Autodesk Inventor part; units mm, degrees
(part 2 of 2)
  arc A454 (149.024, -44.4083) -> (153.7778, -44.1859) centre (149.9853, -14.0418) ccw projected
  arc A455 (153.7778, -44.1859) -> (154.2042, -42.674) centre (0, 0) ccw projected
  arc A456 (154.2042, -42.674) -> (150.2671, -40.0005) centre (135.2203, -66.3945) ccw projected
  arc A457 (150.2671, -40.0005) -> (150.6526, -38.5234) centre (0, 0) ccw projected
  arc A458 (150.6526, -38.5234) -> (155.394, -38.1145) centre (150.4209, -8.1425) ccw projected
  arc A459 (155.394, -38.1145) -> (155.7607, -36.5871) centre (0, 0) ccw projected
  arc A460 (155.7607, -36.5871) -> (151.7217, -34.0702) centre (137.7226, -61.0346) ccw projected
  arc A461 (151.7217, -34.0702) -> (152.0488, -32.5791) centre (0, 0) ccw projected
  arc A462 (152.0488, -32.5791) -> (156.7705, -31.9844) centre (150.6246, -2.2308) ccw projected
  arc A463 (156.7705, -31.9844) -> (157.077, -30.4438) centre (0, 0) ccw projected
  arc A464 (157.077, -30.4438) -> (152.9423, -28.0874) centre (140.0127, -55.5806) ccw projected
  arc A465 (152.9423, -28.0874) -> (153.2107, -26.5846) centre (0, 0) ccw projected
  arc A466 (153.2107, -26.5846) -> (157.9054, -25.8049) centre (150.5961, 3.6845) ccw projected
  arc A467 (157.9054, -25.8049) -> (158.1511, -24.2535) centre (0, 0) ccw projected
  arc A468 (158.1511, -24.2535) -> (153.9271, -22.0613) centre (142.0868, -50.0409) ccw projected
  arc A469 (153.9271, -22.0613) -> (154.1363, -20.5491) centre (0, 0) ccw projected
  arc A470 (154.1363, -20.5491) -> (158.7967, -19.5857) centre (150.3353, 9.594) ccw projected
  arc A471 (158.7967, -19.5857) -> (158.9814, -18.0258) centre (0, 0) ccw projected
  arc A472 (158.9814, -18.0258) -> (154.6745, -16.0011) centre (143.9419, -44.424) ccw projected
  arc A473 (154.6745, -16.0011) -> (154.8242, -14.4819) centre (0, 0) ccw projected
  arc A474 (154.8242, -14.4819) -> (159.4432, -13.3363) centre (149.8427, 15.4887) ccw projected
  arc A475 (159.4432, -13.3363) -> (159.5665, -11.7703) centre (0, 0) ccw projected
  arc A476 (159.5665, -11.7703) -> (155.1835, -9.9163) centre (145.575, -38.7386) ccw projected
  arc A477 (155.1835, -9.9163) -> (155.2734, -8.3923) centre (0, 0) ccw projected
  arc A478 (155.2734, -8.3923) -> (159.8439, -7.0663) centre (149.1191, 21.3596) ccw projected
  arc A479 (159.8439, -7.0663) -> (159.9056, -5.4967) centre (0, 0) ccw projected
  arc A480 (159.9056, -5.4967) -> (155.4532, -3.8162) centre (146.9836, -32.9935) ccw projected
  arc A481 (155.4532, -3.8162) -> (155.4831, -2.2898) centre (0, 0) ccw projected
  arc A482 (155.4831, -2.2898) -> (159.9981, -0.7854) centre (148.1656, 27.1975) ccw projected
  arc A483 (159.9981, -0.7854) -> (159.9981, 0.7854) centre (0, 0) ccw projected
  arc A484 (159.9981, 0.7854) -> (155.4831, 2.2898) centre (148.1656, -27.1975) ccw projected
  arc A485 (155.4831, 2.2898) -> (155.4532, 3.8162) centre (0, 0) ccw projected
  arc A486 (155.4532, 3.8162) -> (159.9056, 5.4967) centre (146.9836, 32.9935) ccw projected
  arc A487 (159.9056, 5.4967) -> (159.8439, 7.0663) centre (0, 0) ccw projected
  arc A488 (159.8439, 7.0663) -> (155.2734, 8.3923) centre (149.1191, -21.3596) ccw projected
  arc A489 (155.2734, 8.3923) -> (155.1835, 9.9163) centre (0, 0) ccw projected
  arc A490 (155.1835, 9.9163) -> (159.5665, 11.7703) centre (145.575, 38.7386) ccw projected
  arc A491 (159.5665, 11.7703) -> (159.4432, 13.3363) centre (0, 0) ccw projected
  arc A492 (159.4432, 13.3363) -> (154.8242, 14.4819) centre (149.8427, -15.4887) ccw projected
  arc A493 (154.8242, 14.4819) -> (154.6745, 16.0011) centre (0, 0) ccw projected
  arc A494 (154.6745, 16.0011) -> (158.9814, 18.0258) centre (143.9419, 44.424) ccw projected
  arc A495 (158.9814, 18.0258) -> (158.7967, 19.5857) centre (0, 0) ccw projected
  arc A496 (158.7967, 19.5857) -> (154.1363, 20.5491) centre (150.3353, -9.594) ccw projected
  arc A497 (154.1363, 20.5491) -> (153.9271, 22.0613) centre (0, 0) ccw projected
  arc A498 (153.9271, 22.0613) -> (158.1511, 24.2535) centre (142.0868, 50.0409) ccw projected
  arc A499 (158.1511, 24.2535) -> (157.9054, 25.8049) centre (0, 0) ccw projected
  arc A500 (157.9054, 25.8049) -> (153.2107, 26.5846) centre (150.5961, -3.6845) ccw projected
  arc A501 (153.2107, 26.5846) -> (152.9423, 28.0874) centre (0, 0) ccw projected
  arc A502 (152.9423, 28.0874) -> (157.077, 30.4438) centre (140.0127, 55.5806) ccw projected
  arc A503 (157.077, 30.4438) -> (156.7705, 31.9844) centre (0, 0) ccw projected
  arc A504 (156.7705, 31.9844) -> (152.0488, 32.5791) centre (150.6246, 2.2308) ccw projected
  arc A505 (152.0488, 32.5791) -> (151.7217, 34.0702) centre (0, 0) ccw projected
  arc A506 (151.7217, 34.0702) -> (155.7607, 36.5871) centre (137.7226, 61.0346) ccw projected
  arc A507 (155.7607, 36.5871) -> (155.394, 38.1145) centre (0, 0) ccw projected
  arc A508 (155.394, 38.1145) -> (150.6526, 38.5234) centre (150.4209, 8.1425) ccw projected
  arc A509 (150.6526, 38.5234) -> (150.2671, 40.0005) centre (0, 0) ccw projected
  arc A510 (150.2671, 40.0005) -> (154.2042, 42.674) centre (135.2203, 66.3945) ccw projected
  arc A511 (154.2042, 42.674) -> (153.7778, 44.1859) centre (0, 0) ccw projected
  arc A512 (153.7778, 44.1859) -> (149.024, 44.4083) centre (149.9853, 14.0418) ccw projected
  arc A513 (149.024, 44.4083) -> (148.5809, 45.8692) centre (0, 0) ccw projected
  arc A514 (148.5809, 45.8692) -> (152.4099, 48.6952) centre (132.5094, 71.6521) ccw projected
  arc A515 (152.4099, 48.6952) -> (151.9245, 50.1891) centre (0, 0) ccw projected
  arc A516 (151.9245, 50.1891) -> (147.1657, 50.2247) centre (149.3183, 19.9193) ccw projected
  arc A517 (147.1657, 50.2247) -> (146.6655, 51.6671) centre (0, 0) ccw projected
  arc A518 (146.6655, 51.6671) -> (150.3806, 54.6412) centre (129.5942, 76.7991) ccw projected
  arc A519 (150.3806, 54.6412) -> (149.837, 56.1149) centre (0, 0) ccw projected
  arc A520 (149.837, 56.1149) -> (145.0804, 55.9637) centre (148.4212, 25.7662) ccw projected
  arc A521 (145.0804, 55.9637) -> (144.524, 57.3853) centre (0, 0) ccw projected
  arc A522 (144.524, 57.3853) -> (148.1195, 60.503) centre (126.4791, 81.8277) ccw projected
  arc A523 (148.1195, 60.503) -> (147.5184, 61.9542) centre (0, 0) ccw projected
  arc A524 (147.5184, 61.9542) -> (142.7714, 61.6164) centre (147.2952, 31.5733) ccw projected
  arc A525 (142.7714, 61.6164) -> (142.1596, 63.015) centre (0, 0) ccw projected
  arc A526 (142.1596, 63.015) -> (145.63, 66.2715) centre (123.1691, 86.7302) ccw projected
  arc A527 (145.63, 66.2715) -> (144.9723, 67.698) centre (0, 0) ccw projected
  arc A528 (144.9723, 67.698) -> (140.2423, 67.174) centre (145.9421, 37.3317) ccw projected
  arc A529 (140.2423, 67.174) -> (139.5761, 68.5476) centre (0, 0) ccw projected
  arc A530 (139.5761, 68.5476) -> (142.9159, 71.9378) centre (119.6691, 91.4989) ccw projected
  arc A531 (142.9159, 71.9378) -> (142.2028, 73.3374) centre (0, 0) ccw projected
  arc A532 (142.2028, 73.3374) -> (137.4969, 72.6281) centre (144.3639, 43.0326) ccw projected
  arc A533 (137.4969, 72.6281) -> (136.7773, 73.9745) centre (0, 0) ccw projected
  arc A534 (136.7773, 73.9745) -> (139.9814, 77.4932) centre (115.9846, 96.1266) ccw projected
  arc A535 (139.9814, 77.4932) -> (139.2139, 78.8637) centre (0, 0) ccw projected
  arc A536 (139.2139, 78.8637) -> (134.5396, 77.9702) centre (142.5632, 48.6671) ccw projected
  arc A537 (134.5396, 77.9702) -> (133.7676, 79.2873) centre (0, 0) ccw projected
  arc A538 (133.7676, 79.2873) -> (136.8312, 82.9291) centre (112.1213, 100.606) ccw projected
  arc A539 (136.8312, 82.9291) -> (136.0104, 84.2684) centre (0, 0) ccw projected
  arc A540 (136.0104, 84.2684) -> (131.3747, 83.1921) centre (140.5426, 54.2266) ccw projected
  arc A541 (131.3747, 83.1921) -> (130.5517, 84.4779) centre (0, 0) ccw projected
  arc A542 (130.5517, 84.4779) -> (133.4699, 88.2371) centre (108.0851, 104.9303) ccw projected
  arc A543 (133.4699, 88.2371) -> (132.5972, 89.5432) centre (0, 0) ccw projected
  arc A544 (132.5972, 89.5432) -> (128.0073, 88.2857) centre (138.3053, 59.7025) ccw projected
  arc A545 (128.0073, 88.2857) -> (127.1344, 89.5382) centre (0, 0) ccw projected
  arc A546 (127.1344, 89.5382) -> (129.9028, 93.4091) centre (103.8822, 109.0928) ccw projected
  arc A547 (129.9028, 93.4091) -> (128.9795, 94.6799) centre (0, 0) ccw projected
  arc A548 (128.9795, 94.6799) -> (124.4426, 93.2432) centre (135.8548, 65.0863) ccw projected
  arc A549 (124.4426, 93.2432) -> (123.5212, 94.4604) centre (0, 0) ccw projected
  arc A550 (123.5212, 94.4604) -> (126.1354, 98.4371) centre (99.5191, 113.0871) ccw projected
  arc A551 (126.1354, 98.4371) -> (125.163, 99.6706) centre (0, 0) ccw projected
  arc A552 (125.163, 99.6706) -> (120.6859, 98.0569) centre (133.1948, 70.3698) ccw projected
  arc A553 (120.6859, 98.0569) -> (119.7174, 99.237) centre (0, 0) ccw projected
  arc A554 (119.7174, 99.237) -> (122.1736, 103.3132) centre (95.0026, 116.907) ccw projected
  arc A555 (122.1736, 103.3132) -> (121.1534, 104.5077) centre (0, 0) ccw projected
  arc A556 (121.1534, 104.5077) -> (116.7432, 102.7194) centre (130.3294, 75.5447) ccw projected
  arc A557 (116.7432, 102.7194) -> (115.7291, 103.8606) centre (0, 0) ccw projected
  arc A558 (115.7291, 103.8606) -> (118.0233, 108.0301) centre (90.3396, 120.5467) ccw projected
  arc A559 (118.0233, 108.0301) -> (116.9571, 109.1835) centre (0, 0) ccw projected
  arc A560 (116.9571, 109.1835) -> (112.6204, 107.2236) centre (127.263, 80.6032) ccw projected
  arc A561 (112.6204, 107.2236) -> (111.5623, 108.324) centre (0, 0) ccw projected
  arc A562 (111.5623, 108.324) -> (113.6911, 112.5804) centre (85.5374, 124.0004) ccw projected
  arc A563 (113.6911, 112.5804) -> (112.5804, 113.6911) centre (0, 0) ccw projected
  arc A564 (112.5804, 113.6911) -> (108.324, 111.5623) centre (124.0004, 85.5374) ccw projected
  arc A565 (108.324, 111.5623) -> (107.2236, 112.6204) centre (0, 0) ccw projected
  arc A566 (107.2236, 112.6204) -> (109.1835, 116.9571) centre (80.6032, 127.263) ccw projected
  arc A567 (109.1835, 116.9571) -> (108.0301, 118.0233) centre (0, 0) ccw projected
  arc A568 (108.0301, 118.0233) -> (103.8606, 115.7291) centre (120.5467, 90.3396) ccw projected
  arc A569 (103.8606, 115.7291) -> (102.7194, 116.7432) centre (0, 0) ccw projected
  arc A570 (102.7194, 116.7432) -> (104.5077, 121.1534) centre (75.5447, 130.3294) ccw projected
  arc A571 (104.5077, 121.1534) -> (103.3132, 122.1736) centre (0, 0) ccw projected
  arc A572 (103.3132, 122.1736) -> (99.237, 119.7174) centre (116.907, 95.0026) ccw projected
  arc A573 (99.237, 119.7174) -> (98.0569, 120.6859) centre (0, 0) ccw projected
  arc A574 (98.0569, 120.6859) -> (99.6706, 125.163) centre (70.3698, 133.1948) ccw projected
  arc A575 (99.6706, 125.163) -> (98.4371, 126.1354) centre (0, 0) ccw projected
  arc A576 (98.4371, 126.1354) -> (94.4604, 123.5212) centre (113.0871, 99.5191) ccw projected
  arc A577 (94.4604, 123.5212) -> (93.2432, 124.4426) centre (0, 0) ccw projected
  arc A578 (93.2432, 124.4426) -> (94.6799, 128.9795) centre (65.0863, 135.8548) ccw projected
  arc A579 (94.6799, 128.9795) -> (93.4091, 129.9028) centre (0, 0) ccw projected
  arc A580 (93.4091, 129.9028) -> (89.5382, 127.1344) centre (109.0928, 103.8822) ccw projected
  arc A581 (89.5382, 127.1344) -> (88.2857, 128.0073) centre (0, 0) ccw projected
  arc A582 (88.2857, 128.0073) -> (89.5432, 132.5972) centre (59.7025, 138.3053) ccw projected
  arc A583 (89.5432, 132.5972) -> (88.2371, 133.4699) centre (0, 0) ccw projected
  arc A584 (88.2371, 133.4699) -> (84.4779, 130.5517) centre (104.9303, 108.0851) ccw projected
  arc A585 (84.4779, 130.5517) -> (83.1921, 131.3747) centre (0, 0) ccw projected
  arc A586 (83.1921, 131.3747) -> (84.2684, 136.0104) centre (54.2266, 140.5426) ccw projected
  arc A587 (84.2684, 136.0104) -> (82.9291, 136.8312) centre (0, 0) ccw projected
  arc A588 (82.9291, 136.8312) -> (79.2873, 133.7676) centre (100.606, 112.1213) ccw projected
  arc A589 (79.2873, 133.7676) -> (77.9702, 134.5396) centre (0, 0) ccw projected
  arc A590 (77.9702, 134.5396) -> (78.8637, 139.2139) centre (48.6671, 142.5632) ccw projected
  arc A591 (78.8637, 139.2139) -> (77.4932, 139.9814) centre (0, 0) ccw projected
  arc A592 (77.4932, 139.9814) -> (73.9745, 136.7773) centre (96.1266, 115.9846) ccw projected
  arc A593 (73.9745, 136.7773) -> (72.6281, 137.4969) centre (0, 0) ccw projected
  arc A594 (72.6281, 137.4969) -> (73.3374, 142.2028) centre (43.0326, 144.3639) ccw projected
  arc A595 (73.3374, 142.2028) -> (71.9378, 142.9159) centre (0, 0) ccw projected
  arc A596 (71.9378, 142.9159) -> (68.5476, 139.5761) centre (91.4989, 119.6691) ccw projected
  arc A597 (68.5476, 139.5761) -> (67.174, 140.2423) centre (0, 0) ccw projected
  arc A598 (67.174, 140.2423) -> (67.698, 144.9723) centre (37.3317, 145.9421) ccw projected
  arc A599 (67.698, 144.9723) -> (66.2715, 145.63) centre (0, 0) ccw projected
  arc A600 (66.2715, 145.63) -> (63.015, 142.1596) centre (86.7302, 123.1691) ccw projected
  arc A601 (63.015, 142.1596) -> (61.6164, 142.7714) centre (0, 0) ccw projected
  arc A602 (61.6164, 142.7714) -> (61.9542, 147.5184) centre (31.5733, 147.2952) ccw projected
  arc A603 (61.9542, 147.5184) -> (60.503, 148.1195) centre (0, 0) ccw projected
  arc A604 (60.503, 148.1195) -> (57.3853, 144.524) centre (81.8277, 126.4791) ccw projected
  arc A605 (57.3853, 144.524) -> (55.9637, 145.0804) centre (0, 0) ccw projected
  arc A606 (55.9637, 145.0804) -> (56.1149, 149.837) centre (25.7662, 148.4212) ccw projected
  arc A607 (56.1149, 149.837) -> (54.6412, 150.3806) centre (0, 0) ccw projected
  arc A608 (54.6412, 150.3806) -> (51.6671, 146.6655) centre (76.7991, 129.5942) ccw projected
  arc A609 (51.6671, 146.6655) -> (50.2247, 147.1657) centre (0, 0) ccw projected
  arc A610 (50.2247, 147.1657) -> (50.1891, 151.9245) centre (19.9193, 149.3183) ccw projected
  arc A611 (50.1891, 151.9245) -> (48.6952, 152.4099) centre (0, 0) ccw projected
  arc A612 (48.6952, 152.4099) -> (45.8692, 148.5809) centre (71.6521, 132.5094) ccw projected
  arc A613 (45.8692, 148.5809) -> (44.4083, 149.024) centre (0, 0) ccw projected
  arc A614 (44.4083, 149.024) -> (44.1859, 153.7778) centre (14.0418, 149.9853) ccw projected
  arc A615 (44.1859, 153.7778) -> (42.674, 154.2042) centre (0, 0) ccw projected
  arc A616 (42.674, 154.2042) -> (40.0005, 150.2671) centre (66.3945, 135.2203) ccw projected
  arc A617 (40.0005, 150.2671) -> (38.5234, 150.6526) centre (0, 0) ccw projected
  arc A618 (38.5234, 150.6526) -> (38.1145, 155.394) centre (8.1425, 150.4209) ccw projected
  arc A619 (38.1145, 155.394) -> (36.5871, 155.7607) centre (0, 0) ccw projected
  arc A620 (36.5871, 155.7607) -> (34.0702, 151.7217) centre (61.0346, 137.7226) ccw projected
  arc A621 (34.0702, 151.7217) -> (32.5791, 152.0488) centre (0, 0) ccw projected
  arc A622 (32.5791, 152.0488) -> (31.9844, 156.7705) centre (2.2308, 150.6246) ccw projected
  arc A623 (31.9844, 156.7705) -> (30.4438, 157.077) centre (0, 0) ccw projected
  arc A624 (30.4438, 157.077) -> (28.0874, 152.9423) centre (55.5806, 140.0127) ccw projected
  arc A625 (28.0874, 152.9423) -> (26.5846, 153.2107) centre (0, 0) ccw projected
  arc A626 (26.5846, 153.2107) -> (25.8049, 157.9054) centre (-3.6845, 150.5961) ccw projected
  arc A627 (25.8049, 157.9054) -> (24.2535, 158.1511) centre (0, 0) ccw projected
  arc A628 (24.2535, 158.1511) -> (22.0613, 153.9271) centre (50.0409, 142.0868) ccw projected
  arc A629 (22.0613, 153.9271) -> (20.5491, 154.1363) centre (0, 0) ccw projected
  arc A630 (20.5491, 154.1363) -> (19.5857, 158.7967) centre (-9.594, 150.3353) ccw projected
  arc A631 (19.5857, 158.7967) -> (18.0258, 158.9814) centre (0, 0) ccw projected
  arc A632 (18.0258, 158.9814) -> (16.0011, 154.6745) centre (44.424, 143.9419) ccw projected
  arc A633 (16.0011, 154.6745) -> (14.4819, 154.8242) centre (0, 0) ccw projected
  arc A634 (14.4819, 154.8242) -> (13.3363, 159.4432) centre (-15.4887, 149.8427) ccw projected
  arc A635 (13.3363, 159.4432) -> (11.7703, 159.5665) centre (0, 0) ccw projected
  arc A636 (11.7703, 159.5665) -> (9.9163, 155.1835) centre (38.7386, 145.575) ccw projected
  arc A637 (9.9163, 155.1835) -> (8.3923, 155.2734) centre (0, 0) ccw projected
  arc A638 (8.3923, 155.2734) -> (7.0663, 159.8439) centre (-21.3596, 149.1191) ccw projected
  arc A639 (7.0663, 159.8439) -> (5.4967, 159.9056) centre (0, 0) ccw projected
  arc A640 (5.4967, 159.9056) -> (3.8162, 155.4532) centre (32.9935, 146.9836) ccw projected
  arc A641 (3.8162, 155.4532) -> (2.2898, 155.4831) centre (0, 0) ccw projected
  arc A642 (2.2898, 155.4831) -> (0.7854, 159.9981) centre (-27.1975, 148.1656) ccw projected
  arc A643 (0.7854, 159.9981) -> (-0.7854, 159.9981) centre (0, 0) ccw projected
  arc A644 (-0.7854, 159.9981) -> (-2.2898, 155.4831) centre (27.1975, 148.1656) ccw projected
  arc A645 (-2.2898, 155.4831) -> (-3.8162, 155.4532) centre (0, 0) ccw projected
  arc A646 (-3.8162, 155.4532) -> (-5.4967, 159.9056) centre (-32.9935, 146.9836) ccw projected
  arc A647 (-5.4967, 159.9056) -> (-7.0663, 159.8439) centre (0, 0) ccw projected
  point P0 (-148.1195, -60.503)
  point P1 (103.3974, 41.0554)
  point P2 (-103.3974, -41.0554)
  dimension "d123" = 22.125
  dimension "d124" = 20
  dimension "d125" = 15
  dimension "d126" = 1
  dimension "d127" = 1
  dimension "d128" = 4
  constraints: 52 end point, 16 symmetric about line, 5 point on line, 3 perpendicular, 1 coincident, 1 horizontal, 1 parallel, 1 vertical
  measures "d123" distance of L3.end L4.end
  measures "d124" distance of L4.end L5.end
  measures "d125" distance of L5.end L6.end
  measures "d126" distance of L10.end L7.end
  measures "d127" distance of L9.start L11.end
  measures "d128" distance of L11.end L12.end
extrude "Extrusion7" cut sketch "Sketch11" along normal mid plane 50 contours A0 L1 L23 L22 L25 L24 A521 A520 A519 A518 A517 A516 A515 A514 A513 A512 A511 A510 A509 A508 A507 A506 A505 A504 A503 A502 A501 A500 A499 A498 A497 A496 A495 A494 A493 A492 A491 A490 A489 A488 A487 A486 A485 A484 A483 A482 A481 A480 A479 A478 A477 A476 A475 A474 A473 A472 A471 A470 A469 A468 A467 A466 A465 A464 A463 A462 A461 A460 A459 A458 A457 A456 A455 A454 A453 A452 A451 A450 A449 A448 A447 A446 A445 A444 A443 A442 A441 A440 A439 A438 A437 A436 A435 A434 A433 A432 A431 A430 A429 A428 A427 A426 A425 A424 A423 A422 A421 A420 A419 A418 A417 A416 A415 A414 A413 A412 A411 A410 A409 A408 A407 A406 A405 A404 A403 A402 A401 A400 A399 A398 A397 A396 A395 A394 A393 A392 A391 A390 A389 A388 A387 A386 A385 A384 A383 A382 A381 A380 A379 A378 A377 A376 A375 A374 A373 A372 A371 A370 A369 A368 A367 A366 A365 A364 A363 A362 A361 A360 A359 A358 A357 A356 A355 A354 A353 A352 A351 A350 A349 A348 A347 A346 A345 A344 A343 A342 A341 A340 A339 A338 A337 A336 A335 A334 A333 A332 A331 A330 A329 A328 A327 A326 A325 A324 A323 A322 A321 A320 A319 A318 A317 A316 A315 A314 A313 A312 A311 A310 A309 A308 A307 A306 A305 A304 A303 A302 A301 A300 A299 A298 A297 A296 A295 A294 A293 A292 A291 A290 A289 A288 A287 A286 A285 A284 A283 A282 A281 A280 A279 A278 A277 A276 A275 A274 A273 A272 A271 A270 A269 A268 A267 A266 A265 A264 A263 A262 A261 A260 A259 A258 A257 A256 A255 A254 A253 A252 A251 A250 A249 A248 A247 A246 A245 A244 A243 A242 A241 A240 A239 A238 A237 A236 A235 A234 A233 A232 A231 A230 A229 A228 A227 A226 A225 A224 A223 A222 A221 A220 A219 A218 A217 A216 A215 A214 A213 A212 A211 A210 A209 A208 A207 A206 A205 A204 A203 A2 L3 L20 L19 L6 L7 | L3 L9 L11 L12 L13 | L7 L6 L5 L3 | L3 L14 L15 L18 L11 L9 | L5 L19 L20 L3 | L3 L17 L16 L15 L14 | L34 L35 L36 L37 | L38 L39 L40 L41 | L42 L43 L44 L45 | L46 L47 L48 L49
sketch "Sketch12" plane through (0, 0, 15) normal (0, 0, 1) x (1, 0, 0)
  point P0 (0, 0)
  point P1 (0, 0)
  constraints: 1 coincident
equation "\"d0\" = da_da"
equation "\"d3\" = da_d"
equation "\"da_da\" = 320"
equation "\"da_d\" = 320"
body "Solid1"
body "Srf1"
